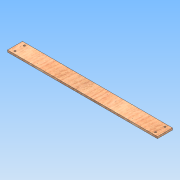
# Autodesk Inventor part: Top_End Piece 1
Saved by Autodesk Inventor 2018.1 (Build 221171000, 171)
## iProperties
Created: 2019-03-24
Part Number: Top_End Piece 1
Material: Wood (Birch)
Document SubType Name: Modeling
Designer: James
Density: 0.55 g/cm^3
Appearance: Birch - Natural Polished
Author: James
Autodesk Inventor part; units mm, degrees
ref_plane "YZ Plane" through (0, 0, 0) normal (1, 0, 0) x (0, 1, 0)
ref_plane "XZ Plane" through (0, 0, 0) normal (0, 1, 0) x (-1, 0, 0)
ref_plane "XY Plane" through (0, 0, 0) normal (0, 0, 1) x (1, 0, 0)
sketch "Sketch1" plane through (0, 0, 0) normal (0, 0, 1) x (1, 0, 0)
  line L0 (0, 0) -> (400, 0)
  line L1 (400, 0) -> (400, 40)
  line L2 (400, 40) -> (0, 40)
  line L3 (0, 40) -> (0, 0)
  dimension "d0" = 400
  dimension "d1" = 40
  constraints: 8 end point, 2 parallel, 1 horizontal, 1 perpendicular
  measures "d0" distance of L2.end L1.end
  measures "d1" distance of L1.end L0.end
extrude "Extrusion1" add sketch "Sketch1" along normal blind 5
sketch "Sketch2" plane through (0, 0, 5) normal (0, 0, 1) x (1, 0, 0)
  line L0 (400, 40) -> (0, 40) projected
  line L1 (0, 40) -> (0, 0) projected
  line L2 (0, 0) -> (400, 0) projected
  line L3 (400, 0) -> (400, 40) projected
  point P0 (12.5, 32.5)
  point P1 (12.5, 7.5)
  point P2 (387.5, 32.5)
  point P3 (387.5, 7.5)
  dimension "d4" = 7.5
  dimension "d5" = 12.5
  dimension "d6" = 7.5
  dimension "d7" = 12.5
  constraints: 2 horizontal alignment, 2 vertical alignment
  measures "d4" distance from line of L0 point (12.5, 32.5)
  measures "d5" distance from line of L1 point (12.5, 32.5)
  measures "d6" distance from line of L2 point (12.5, 7.5)
  measures "d7" distance from line of L3 point (387.5, 32.5)
hole "Hole1" at (12.5, 32.5, 5) at (12.5, 7.5, 5) at (387.5, 32.5, 5) at (387.5, 7.5, 5) direction (0, 0, -1) diameter 4.5 end through all clearance for "Flat Head Machine Screw" size "M4" standard "Ansi Metric M Profile"
equation "\"d6\" = d4"
equation "\"d7\" = d5"
body "Solid1"
